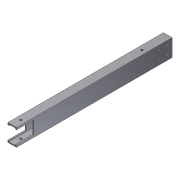
# Autodesk Inventor part: Frame_UpperRollerMount
Saved by Autodesk Inventor 2012 (Build 160160000, 160)
## iProperties
Created: 2012-01-14
Part Number: Frame_UpperRollerMount
Material: Default
Document SubType Name: Modeling
Designer: JesseK
Density: 1 g/cm^3
Mass: 189.645 g
Surface Area: 1216.27 cm^2
Volume: 189.645 cm^3
Author: JesseK
Autodesk Inventor part; units mm, degrees
ref_plane "YZ Plane" through (0, 0, 0) normal (1, 0, 0) x (0, 1, 0)
ref_plane "XZ Plane" through (0, 0, 0) normal (0, 1, 0) x (-1, 0, 0)
ref_plane "XY Plane" through (0, 0, 0) normal (0, 0, 1) x (1, 0, 0)
sketch "Sketch1" plane through (0, 0, 0) normal (0, 0, 1) x (1, 0, 0)
  line L0 (0, 0) -> (25.4, 0)
  line L1 (25.4, 0) -> (25.4, 50.8)
  line L2 (25.4, 50.8) -> (0, 50.8)
  line L3 (0, 50.8) -> (0, 0)
  dimension "d0" = 25.4
  dimension "d1" = 50.8
  constraints: 8 end point, 2 parallel, 1 horizontal, 1 perpendicular
  measures "d0" distance of L0.start L0.end
  measures "d1" distance of L2.end L0.start
extrude "Extrusion1" add sketch "Sketch1" along normal blind 457.2
shell "Shell1" thickness 3.175 removed faces 2 at (8.4667, 33.8667, 0) at (8.4667, 33.8667, 457.2)
sketch "Sketch2" plane through (25.4, 0, 0) normal (1, 0, 0) x (0, 0, -1)
  line L0 (0, 50.8) -> (-457.2, 50.8) projected
  line L1 (-457.2, 44.45) -> (-406.4, 44.45)
  line L2 (-406.4, 44.45) -> (-406.4, 6.35)
  line L3 (-406.4, 6.35) -> (-457.2, 6.35)
  line L4 (-457.2, 6.35) -> (-457.2, 44.45)
  line L5 (0, 0) -> (0, 50.8) projected
  dimension "d24" = 38.1
  dimension "d26" = 6.35
  dimension "d27" = 406.4
  dimension "d28" = 50.8
  constraints: 8 end point, 2 parallel, 1 horizontal, 1 perpendicular
  measures "d24" distance between parallel lines of L3 L1
  measures "d26" distance between parallel lines of L0 L1
  measures "d27" distance between parallel lines of L5 L2
  measures "d28" distance between parallel lines of L4 L2
extrude "Extrusion2" cut sketch "Sketch2" against normal through all
sketch "Sketch3" plane through (0, 50.8, 0) normal (0, 1, 0) x (1, 0, 0)
  line L0 (0, -457.2) -> (25.4, -457.2) projected
  line L1 (25.4, 0) -> (25.4, -457.2) projected
  line L2 (25.4, 0) -> (0, 0) projected
  line L3 (0, 0) -> (0, -457.2) projected
  circle A0 centre (12.7, -76.2) radius 3.175
  circle A1 centre (12.7, -431.8) radius 3.175
  dimension "d15" = 12.7
  dimension "d16" = 76.2
  dimension "d17" = 6.35
  dimension "d18" = 12.7
  dimension "d19" = 6.35
  dimension "d20" = 25.4
  constraints: 2 centre point
  measures "d15" distance from line of L3 A0.centre
  measures "d16" distance from line of L2 A0.centre
  measures "d17" diameter of A0
  measures "d18" distance from line of L1 A1.centre
  measures "d19" diameter of A1
  measures "d20" distance from line of L0 A1.centre
extrude "Extrusion3" cut sketch "Sketch3" against normal through all contours A0 | A1
sketch "Sketch4" plane through (25.4, 0, 0) normal (1, 0, 0) x (0, 0, -1)
  line L0 (0, 0) -> (0, 50.8) projected
  line L1 (0, 50.8) -> (-457.2, 50.8) projected
  circle A0 centre (-38.1, 38.1) radius 2.3813
  circle A1 centre (-12.7, 38.1) radius 2.3813
  circle A2 centre (-38.1, 12.7) radius 2.3813
  circle A3 centre (-12.7, 12.7) radius 2.3813
  line L2 (-38.1, 38.1) -> (-12.7, 38.1) construction
  line L3 (-12.7, 38.1) -> (-12.7, 12.7) construction
  line L4 (-12.7, 12.7) -> (-38.1, 12.7) construction
  line L5 (-38.1, 12.7) -> (-38.1, 38.1) construction
  dimension "d29" = 4.7625
  dimension "d30" = 12.7
  dimension "d31" = 25.4
  dimension "d32" = 25.4
  dimension "d33" = 12.7
  constraints: 8 end point, 4 centre point, 3 coincident, 3 equal radius, 2 parallel, 1 horizontal, 1 perpendicular
  measures "d29" diameter of A1
  measures "d30" distance between parallel lines of L1 L2
  measures "d31" distance of L2.end L3.end
  measures "d32" distance of L3.end L4.end
  measures "d33" distance between parallel lines of L0 L3
extrude "Extrusion4" cut sketch "Sketch4" against normal through all
body "Solid1"
